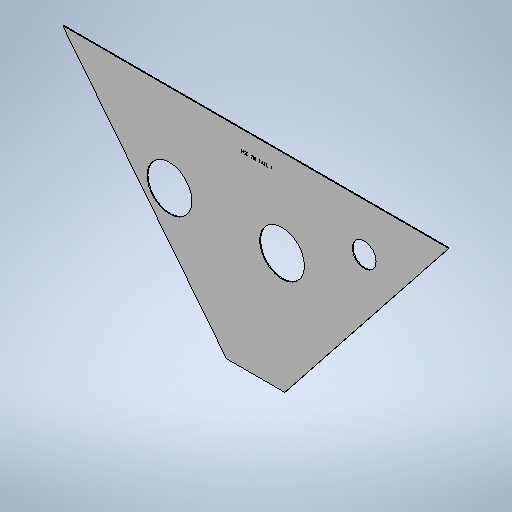
# Autodesk Inventor part: MSC 701 FACE 1
Saved by Autodesk Inventor 2025.1 (Build 291241020, 241B)
## iProperties
Created: 2024-06-08
Part Number: MSC 701 FACE 1
Material: Stainless Steel
Document SubType Name: Sheet Metal
Designer: admin
Density: 8 g/cm^3
Sheet Metal Rule: AISI304 3mm Die 32
Appearance: Default
Stock Number: МОО 701 морда 1
Flat Pattern Width: 139.759 cm
Flat Pattern Length: 98.1911 cm
Flat Pattern Area: 13723.1 cm^2
Sheet Metal Width: 1397.594 mm
Sheet Metal Length: 981.911 mm
Sheet Metal Area: 1372313.037 mm^2
Mass: 9882.34 g
Surface Area: 12453.9 cm^2
Volume: 1235.29 cm^3
Author: admin
Autodesk Inventor part; units mm, degrees
ref_plane "YZ Plane" through (0, 0, 0) normal (1, 0, 0) x (0, 1, 0)
ref_plane "XZ Plane" through (0, 0, 0) normal (0, 1, 0) x (-1, 0, 0)
ref_plane "XY Plane" through (0, 0, 0) normal (0, 0, 1) x (1, 0, 0)
sketch "Sketch1" plane through (0, 0, 0) normal (0, 1, 0) x (-1, 0, 0)
  line L0 (0, 780) -> (0, 0)
  line L1 (727.158, 778) -> (727.158, 780)
  line L2 (727.158, 780) -> (0, 780)
  line L3 (727.158, 778) -> (110, 0)
  line L4 (110, 0) -> (0, 0)
  point P0 (0, 678)
  dimension "d1" = 727.158
  dimension "d2" = 2
  dimension "d5" = 128.424
  dimension "d6" = 110
  dimension "d9" = 780
  measures "d1" distance of L1.end L0.start
  measures "d2" distance of L1.start L1.end
  measures "d5" angle of L4 L3
  measures "d6" distance of L0.end L3.end
  measures "d9" distance of L0.start L0.end
extrude "Plate1" add sketch "Sketch1" along normal blind 3
mirror "Mirror1" about plane through (0, 0, 0) normal (1, 0, 0) of "Plate1"
sketch "Sketch2" plane through (0, 0, 0) normal (0, -1, 0) x (1, 0, 0)
  line L0 (-110, 0) -> (110, 0) construction
  line L1 (-110, 0) -> (-727.158, 778) construction
  circle A0 centre (-325, 450) radius 84.5
  line L2 (110, 0) -> (727.158, 778) construction
  circle A1 centre (100, 450) radius 84.5
  circle A2 centre (410, 600) radius 45
  line L3 (-110, 0) -> (110, 0) construction
  line L4 (-240.5, 450) -> (-240.5, 164.5105) construction
  line L5 (365, 600) -> (365, 0) construction
  line L6 (-325, 534.5) -> (365, 534.5) construction
  line L7 (-325, 365.5) -> (365, 365.5) construction
  line L8 (100, 534.5) -> (365, 534.5) construction
  line L9 (410, 555) -> (365, 555) construction
  line L10 (-727.158, 780) -> (727.158, 780) projected
  line L11 (-727.158, 778) -> (-727.158, 780) projected
  line L12 (727.158, 778) -> (727.158, 780) projected
  point P0 (0, 0)
  point P1 (0, 0)
  point P2 (0, 0)
  point P3 (0, 0)
  point P4 (0, 0)
  point P5 (0, 0)
  point P6 (0, 0)
  dimension "d13" = 169
  dimension "d16" = 450
  dimension "d17" = 450
  dimension "d18" = 325
  dimension "d19" = -169
  dimension "d20" = 90
  dimension "d23" = 410
  dimension "d24" = 600
  dimension "d29" = 100
  constraints: 12 end point, 5 point on circle, 5 point on line, 5 tangent, 3 horizontal, 3 perpendicular, 2 centre point, 1 midpoint, 1 vertical, 1 vertical alignment, 10 other
  measures "d13" diameter of A0
  measures "d16" distance from line of L0 point (100, 450)
  measures "d17" distance from line of L0 A0.centre
  measures "d18" horizontal distance of A0.centre point (0, 0)
  measures "d19" distance between parallel lines of L8 L7
  measures "d20" diameter of A2
  measures "d23" horizontal distance of point (0, 0) A2.centre
  measures "d24" distance from line of L0 A2.centre
  measures "d29" horizontal distance of point (0, 0) point (100, 450)
extrude "Extrusion1" cut sketch "Sketch2" against normal through all
sketch "Sketch3" plane through (0, 0, 0) normal (0, -1, 0) x (1, 0, 0)
  line L0 (-53.9958, 701.8167) -> (-53.9958, 713.8167) construction
  line L1 (-53.9958, 713.8167) -> (56.0042, 713.8167) construction
  line L2 (56.0042, 713.8167) -> (56.0042, 701.8167) construction
  line L3 (56.0042, 701.8167) -> (-53.9958, 701.8167) construction
  point P0 (0, 0)
  point P1 (1.0042, 701.8167)
  dimension "d25" = 12
  dimension "d26" = 110
  constraints: 1 midpoint, 2 other
  measures "d25" distance of L1.end L2.end
  measures "d26" distance between parallel lines of L0 L2
mark "Mark1"
equation "\"d3\" = Thickness"
equation "\"Thickness\" = 3"
body "Solid1"
